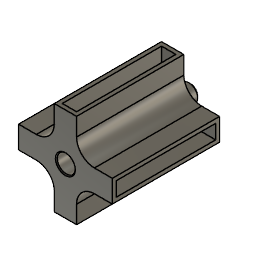
Shoe Rack Bracket_v1 (Autodesk Fusion 360 design; units mm, degrees)
part number: 2026-01-17-13-48-35-251
Autodesk Fusion 360 part; units mm, degrees
sketch "Sketch1" plane through (0, 0, 0) normal (0, 1, 0) x (1, 0, 0)
sketch "Sketch2" plane through (0, 0, 0) normal (0, 1, 0) x (1, 0, 0)
  line L0 (-39.0176, 15.875) -> (-15.875, 15.875)
  line L1 (-15.875, 15.875) -> (-15.875, 66.675)
  line L2 (-15.875, 66.675) -> (15.875, 66.675)
  line L3 (15.875, 66.675) -> (15.875, 15.875)
  line L4 (15.875, 15.875) -> (66.675, 15.875)
  line L5 (66.675, 15.875) -> (66.675, -15.875)
  line L6 (66.675, -15.875) -> (15.875, -15.875)
  line L7 (15.875, -15.875) -> (15.875, -66.675)
  line L8 (15.875, -66.675) -> (-15.875, -66.675)
  line L9 (-15.875, -66.675) -> (-15.875, -15.875)
  line L10 (-15.875, -15.875) -> (-66.675, -15.875)
  line L11 (-66.675, -15.875) -> (-66.675, 15.875)
  line L12 (-66.675, 15.875) -> (-39.0176, 15.875)
  line L13 (1.75, 0) -> (22.5, 0)
  line L14 (0, -1.75) -> (0, -22.5)
  dimension "d1" = 31.75
  dimension "d2" = 31.75
  dimension "d7" = 50.8
  dimension "d8" = 50.8
  constraint horizontal L0
  constraint perpendicular L0 L1
  constraint perpendicular L1 L2
  constraint perpendicular L2 L3
  constraint perpendicular L3 L4
  constraint perpendicular L4 L5
  constraint perpendicular L5 L6
  constraint perpendicular L6 L7
  constraint perpendicular L5 L8
  constraint perpendicular L6 L9
  constraint perpendicular L9 L10
  constraint perpendicular L10 L11
  constraint perpendicular L11 L12
  constraint collinear L1 L9
  constraint collinear L3 L7
  constraint collinear L6 L10
  constraint collinear L4 L12
  constraint equal L3 L7
  constraint equal L6 L10
  constraint symmetric L2 L8 L13
  measures "d1" distance of L7 L9
  measures "d2" distance of L10 L12
  measures "d7" distance of L6 L8
  measures "d8" distance of L5 L7
extrude "Extrude1" add sketch "Sketch2" along normal blind 152.4
sketch "Sketch3" plane through (-66.675, 0, 0) normal (-1, 0, 0) x (0, -1, 0)
  line L0 (0, -15.875) -> (0, 15.875)
  line L1 (0, 15.875) -> (-152.4, 15.875)
  line L2 (-152.4, 15.875) -> (-152.4, -15.875)
  line L3 (-152.4, -15.875) -> (0, -15.875)
  line L4 (-146.685, 10.16) -> (-5.715, 10.16)
  line L5 (-5.715, 10.16) -> (-5.715, -10.16)
  line L6 (-5.715, -10.16) -> (-146.685, -10.16)
  line L7 (-146.685, -10.16) -> (-146.685, 10.16)
  dimension "d11" = 140.97
  dimension "d12" = 20.32
  dimension "d13" = 5.715
  dimension "d14" = 5.715
  constraint horizontal L4
  constraint vertical L5
  constraint horizontal L6
  constraint vertical L7
  measures "d11" distance of L5 L7
  measures "d12" distance of L4 L6
  measures "d13" distance of L1 L4
  measures "d14" distance of L2 L7
extrude "Extrude2" cut sketch "Sketch3" against normal blind 50.8 contours L4 L5 L6 L7
mirror "Mirror1" about plane through (0, 0, 0) normal (1, 0, 0) of "Extrude2"
fillet "Fillet1" radius 25.4 1 edges at (15.875, 76.2, 15.875)
fillet "Fillet1" radius 25.4 3 edges at (-15.875, 76.2, 15.875) (-15.875, 76.2, -15.875) (15.875, 76.2, -15.875)
sketch "Sketch4" plane through (0, 0, 66.675) normal (0, 0, 1) x (-1, 0, 0)
  line L0 (15.875, 0) -> (-15.875, 0)
  line L1 (-15.875, 0) -> (-15.875, -152.4)
  line L2 (-15.875, -152.4) -> (15.875, -152.4)
  line L3 (15.875, -152.4) -> (15.875, 0)
  line L4 (10.16, -146.685) -> (-10.16, -146.685)
  line L5 (-10.16, -146.685) -> (-10.16, -5.715)
  line L6 (-10.16, -5.715) -> (10.16, -5.715)
  line L7 (10.16, -5.715) -> (10.16, -146.685)
  dimension "d24" = 5.715
  dimension "d25" = 5.715
  dimension "d26" = 5.715
  dimension "d27" = 5.715
  constraint horizontal L4
  constraint vertical L5
  constraint horizontal L6
  constraint vertical L7
  measures "d24" distance of L2 L4
  measures "d25" distance of L0 L6
  measures "d26" distance of L3 L7
  measures "d27" distance of L1 L5
extrude "Extrude3" cut sketch "Sketch4" against normal blind 50.8 contours L4 L5 L6 L7
mirror "Mirror2" about plane through (0, 0, 0) normal (0, 0, 1) of "Extrude3"
sketch "Sketch6" plane through (0, 152.4, 0) normal (0, 1, 0) x (-1, 0, 0)
  line L0 (66.675, -15.875) -> (66.675, 15.875)
  line L1 (66.675, 15.875) -> (41.275, 15.875)
  arc A0 (15.875, 41.275) -> (41.275, 15.875) centre (41.275, 41.275) ccw
  line L2 (15.875, 41.275) -> (15.875, 66.675)
  line L3 (15.875, 66.675) -> (-15.875, 66.675)
  line L4 (-15.875, 66.675) -> (-15.875, 41.275)
  arc A1 (-41.275, 15.875) -> (-15.875, 41.275) centre (-41.275, 41.275) ccw
  line L5 (-41.275, 15.875) -> (-66.675, 15.875)
  line L6 (-66.675, 15.875) -> (-66.675, -15.875)
  line L7 (-66.675, -15.875) -> (-41.275, -15.875)
  arc A2 (-15.875, -41.275) -> (-41.275, -15.875) centre (-41.275, -41.275) ccw
  line L8 (-15.875, -41.275) -> (-15.875, -66.675)
  line L9 (-15.875, -66.675) -> (15.875, -66.675)
  line L10 (15.875, -66.675) -> (15.875, -41.275)
  arc A3 (41.275, -15.875) -> (15.875, -41.275) centre (41.275, -41.275) ccw
  line L11 (41.275, -15.875) -> (66.675, -15.875)
  circle A4 centre (0, 0) radius 12.7
  dimension "d32" = 25.4
  constraint coincident A4.centre origin
  measures "d32" diameter of A4
extrude "Extrude4" add sketch "Sketch6" along normal blind 25.4 contours A4
chamfer "Chamfer1" distance 2.54 angle 45 1 edges at (11.8406, 177.8, -4.5925)
sketch "Sketch7" plane through (0, 0, 0) normal (0, -1, 0) x (1, 0, 0)
  line L0 (-66.675, 15.875) -> (-66.675, -15.875)
  line L1 (-66.675, -15.875) -> (-41.275, -15.875)
  arc A0 (-15.875, -41.275) -> (-41.275, -15.875) centre (-41.275, -41.275) ccw
  line L2 (-15.875, -41.275) -> (-15.875, -66.675)
  line L3 (-15.875, -66.675) -> (15.875, -66.675)
  line L4 (15.875, -66.675) -> (15.875, -41.275)
  arc A1 (41.275, -15.875) -> (15.875, -41.275) centre (41.275, -41.275) ccw
  line L5 (41.275, -15.875) -> (66.675, -15.875)
  line L6 (66.675, -15.875) -> (66.675, 15.875)
  line L7 (66.675, 15.875) -> (41.275, 15.875)
  arc A2 (15.875, 41.275) -> (41.275, 15.875) centre (41.275, 41.275) ccw
  line L8 (15.875, 41.275) -> (15.875, 66.675)
  line L9 (15.875, 66.675) -> (-15.875, 66.675)
  line L10 (-15.875, 66.675) -> (-15.875, 41.275)
  arc A3 (-41.275, 15.875) -> (-15.875, 41.275) centre (-41.275, 41.275) ccw
  line L11 (-41.275, 15.875) -> (-66.675, 15.875)
  circle A4 centre (0, 0) radius 12.827
  dimension "d36" = 25.654
  constraint coincident A4.centre origin
  measures "d36" diameter of A4
extrude "Extrude5" cut sketch "Sketch7" against normal blind 27.94 contours A4
chamfer "Chamfer2" distance 1.27 angle 45 1 edges at (-11.959, 0, 4.6384)
